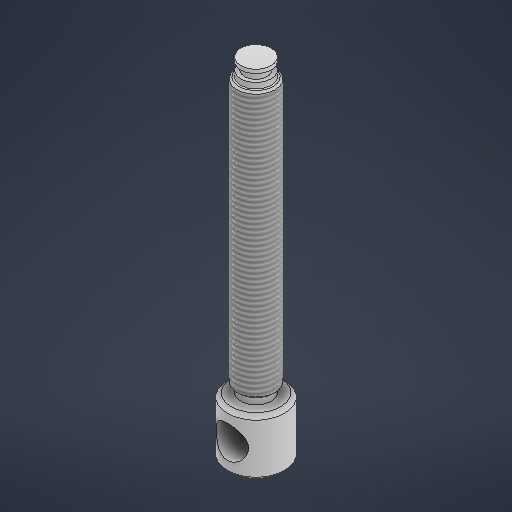
# Autodesk Inventor part: menetesorso
Saved by Autodesk Inventor 2026.1 (Build 301233000, 233)
## iProperties
Created: 2025-09-15
Part Number: menetesorso
Material: Generic
Document SubType Name: Modeling
Designer: student
Density: 1 g/cm^3
Appearance: Default
Author: student
Autodesk Inventor part; units mm, degrees
ref_plane "YZ Plane" through (0, 0, 0) normal (1, 0, 0) x (0, 1, 0)
ref_plane "XZ Plane" through (0, 0, 0) normal (0, 1, 0) x (-1, 0, 0)
sketch "Sketch1" plane through (0, 0, 0) normal (0, 1, 0) x (-1, 0, 0)
  circle A0 centre (0, 0) radius 15
  dimension "d0" = 30
  constraints: 1 centre point, 1 coincident
  measures "d0" diameter of A0
extrude "Extrusion1" add sketch "Sketch1" along normal blind 30
sketch "Sketch2" plane through (0, 30, 0) normal (0, 1, 0) x (1, 0, 0)
  circle A0 centre (0, 0) radius 8
  dimension "d3" = 16
  constraints: 1 centre point, 1 coincident
  measures "d3" diameter of A0
extrude "Extrusion2" add sketch "Sketch2" along normal blind 4
sketch "Sketch3" plane through (0, 34, 0) normal (0, 1, 0) x (1, 0, 0)
  circle A0 centre (0, 0) radius 15 projected
  circle A1 centre (0, 0) radius 10
  dimension "d6" = 20
  constraints: 1 centre point, 1 coincident
  measures "d6" diameter of A1
extrude "Extrusion3" add sketch "Sketch3" along normal blind 140 contours A1
sketch "Sketch4" plane through (0, 174, 0) normal (0, 1, 0) x (1, 0, 0)
  circle A0 centre (0, 0) radius 10 projected
  circle A1 centre (0, 0) radius 8
  dimension "d9" = 16
  constraints: 1 centre point, 1 coincident
  measures "d9" diameter of A1
extrude "Extrusion4" add sketch "Sketch4" along normal blind 3 contours A1
sketch "Sketch5" plane through (0, 177, 0) normal (0, 1, 0) x (1, 0, 0)
  point P0 (0, 0)
sketch "Sketch6" plane through (0, 0, 0) normal (1, 0, 0) x (0, 1, 0)
  line L0 (177, -8) -> (177, 8) projected
  line L1 (177, 0) -> (183, 0)
  line L2 (0, 0) -> (-184.47, 0)
  line L3 (0, -15) -> (0, 15) projected
  line L4 (0, 0) -> (184.47, 0)
  line L5 (184.47, 0) -> (161.97, 0)
  circle A0 centre (161.97, 0) radius 22.5
  line L6 (177, 0) -> (177, 6)
  line L7 (177, 6) -> (181, 6)
  line L8 (181, 6) -> (181, 8)
  line L9 (181, 8) -> (182.9997, 8)
  dimension "d12" = 6
  dimension "d14" = 184.47
  dimension "d15" = 22.5
  dimension "d16" = 6
  dimension "d17" = 4
  dimension "d18" = 2
  constraints: 14 end point, 3 perpendicular, 2 horizontal, 2 point on circle, 2 point on line, 1 centre point, 1 coincident, 1 midpoint, 1 vertical, 3 other
  measures "d12" distance of L1.start L1.end
  measures "d14" distance of L4.start L4.end
  measures "d15" distance of L4.end L5.end
  measures "d16" distance of L1.start L6.end
  measures "d17" distance of L6.end L7.end
  measures "d18" distance of L7.end L8.end
revolve "Revolution1" add sketch "Sketch6" angle 360 about axis through (0, 0, 0) along (0, 1, 0) contours L0 L7 L8 L9 A0 L4 L1
chamfer "Chamfer1" distance 2 angle 45 2 edges at (15, 0, 0) (15, 30, 0)
ref_plane "Work Plane1" through (0, 0, 15) normal (0, 0, 1) x (1, 0, 0)
sketch "Sketch7" plane through (0, 0, 15) normal (0, 0, 1) x (1, 0, 0)
  line L0 (0, 0) -> (0, 15)
  circle A0 centre (0, 15) radius 8.5
  dimension "d23" = 15
  dimension "d24" = 17
  constraints: 2 end point, 1 centre point, 1 coincident, 1 vertical
  measures "d23" distance of L0.start L0.end
  measures "d24" diameter of A0
extrude "Extrusion5" cut sketch "Sketch7" against normal through all
thread "Thread1" size "M20x2.5" class "6g" standard "ANSI Metric M Profile" full length
chamfer "Chamfer2" distance 1 angle 45 1 edges at (-10, 174, 0)
chamfer "Chamfer3" distance 1 angle 45 1 edges at (-10, 34, 0)
body "Solid1"
